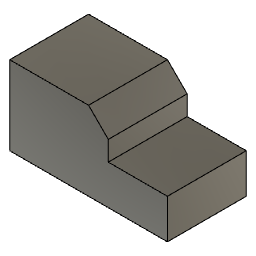
Simple Block (Autodesk Fusion 360 design; units mm, degrees)
Autodesk Fusion 360 part; units mm, degrees
sketch "Sketch1" plane through (0, 0, 0) normal (0, 0, 1) x (1, 0, 0)
  line L0 (25.4, -12.7) -> (-25.4, -12.7)
  line L1 (-25.4, -12.7) -> (-25.4, 12.7)
  line L2 (-25.4, 12.7) -> (25.4, 12.7)
  line L3 (25.4, 12.7) -> (25.4, -12.7)
  line L4 (25.4, -12.7) -> (-25.4, 12.7) construction
  line L5 (-25.4, -12.7) -> (25.4, 12.7) construction
  dimension "d1" = 50.8
  dimension "d2" = 25.4
  constraint horizontal L0
  constraint perpendicular L0 L1
  constraint parallel L0 L2
  constraint parallel L1 L3
  constraint coincident L4 origin
  constraint coincident L5 origin
  measures "d1" distance of L1.end L2.end
  measures "d2" distance of L0.end L1.end
extrude "Extrude1" add sketch "Sketch1" along normal blind 25.4
sketch "Sketch2" plane through (0, -12.7, 0) normal (0, -1, 0) x (1, 0, 0)
  line L0 (-25.4, 0) -> (25.4, 0)
  line L1 (25.4, 0) -> (25.4, 25.4)
  line L2 (25.4, 25.4) -> (-25.4, 25.4)
  line L3 (-25.4, 25.4) -> (-25.4, 0)
  line L4 (25.4, 25.4) -> (6.35, 25.4)
  line L5 (6.35, 25.4) -> (6.35, 12.7)
  line L6 (6.35, 12.7) -> (25.4, 12.7)
  line L7 (25.4, 12.7) -> (25.4, 25.4)
  dimension "d5" = 19.05
  dimension "d6" = 12.7
  constraint horizontal L4
  constraint vertical L5
  constraint horizontal L6
  constraint vertical L7
  constraint coincident L1.end L2.start
  measures "d5" distance of L1.end L4.end
  measures "d6" distance of L1.end L6.end
extrude "Extrude2" cut sketch "Sketch2" against normal through all contours L1 L2 L4 L5 L6 L7
chamfer "Chamfer1" distance 6.35 angle 45 1 edges at (6.35, 0, 25.4)
